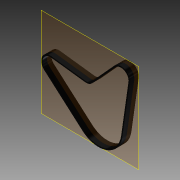
# Autodesk Inventor part: 290 mm Belt
Saved by Autodesk Inventor 2013 (Build 170138000, 138)
## iProperties
Created: 2013-06-27
Part Number: 290 mm Belt
Material: Generic
Document SubType Name: Modeling
Designer: mvarma
Density: 1 g/cm^3
Author: mvarma
Autodesk Inventor part; units mm, degrees
ref_plane "YZ Plane" through (0, 0, 0) normal (1, 0, 0) x (0, 1, 0)
ref_plane "XZ Plane" through (0, 0, 0) normal (0, 1, 0) x (-1, 0, 0)
ref_plane "XY Plane" through (0, 0, 0) normal (0, 0, 1) x (1, 0, 0)
sketch "Sketch1" plane through (0, 0, 0) normal (0, 0, 1) x (1, 0, 0)
  line L0 (84.9408, 79.3264) -> (123.4503, 45.7166)
  line L1 (168.5483, 110.2412) -> (161.1682, 59.6633)
  line L2 (90.9184, 92.6811) -> (125.2091, 88.4019)
  line L3 (132.0626, 90.936) -> (155.3205, 116.4945)
  arc A0 (90.9184, 92.6811) -> (84.9408, 79.3264) centre (89.9711, 85.09) ccw
  arc A1 (128.9448, 88.8334) -> (132.0626, 90.936) centre (126.192, 96.2783) ccw
  arc A2 (125.2091, 88.4019) -> (128.9448, 88.8334) centre (126.192, 96.2783) ccw
  arc A3 (123.4503, 45.7166) -> (161.1682, 59.6633) centre (138.5082, 62.9697) ccw
  arc A4 (168.5483, 110.2412) -> (155.3205, 116.4945) centre (160.9785, 111.3458) ccw
  line L4 (84.1057, 78.3696) -> (122.6152, 44.7598)
  arc A5 (122.6152, 44.7598) -> (162.4249, 59.4799) centre (138.5082, 62.9697) ccw
  line L5 (162.4249, 59.4799) -> (169.805, 110.0578)
  arc A6 (169.805, 110.0578) -> (154.3812, 117.3492) centre (160.9785, 111.3458) ccw
  line L6 (154.3812, 117.3492) -> (131.1233, 91.7908)
  arc A7 (128.5043, 90.0246) -> (131.1233, 91.7908) centre (126.192, 96.2783) ccw
  arc A8 (125.3663, 89.6621) -> (128.5043, 90.0246) centre (126.192, 96.2783) ccw
  line L7 (125.3663, 89.6621) -> (91.0757, 93.9413)
  arc A9 (91.0757, 93.9413) -> (84.1057, 78.3696) centre (89.9711, 85.09) ccw
  point P0 (0, 0)
  dimension "d1" = 1.27
  constraints: 20 point on circle, 16 end point, 10 centre point, 4 tangent, 30 other
  measures "d1" distance between parallel lines of L7 L2
extrude "Extrusion1" add sketch "Sketch1" along normal blind 9
ref_plane "Work Plane1" through (0, 0, 4.5) normal (0, 0, 1) x (1, 0, 0)
body "Solid1"
